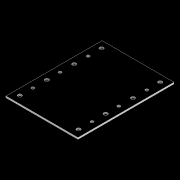
# Autodesk Inventor part: Placa
Saved by Autodesk Inventor 2020 (Build 240168000, 168)
## iProperties
Created: 2020-02-12
Part Number: Placa
Material: Generic
Document SubType Name: Modeling
Designer: PEDRO
Density: 1 g/cm^3
Appearance: Default
Author: PEDRO
Autodesk Inventor part; units mm, degrees
ref_plane "YZ Plane" through (0, 0, 0) normal (1, 0, 0) x (0, 1, 0)
ref_plane "XZ Plane" through (0, 0, 0) normal (0, 1, 0) x (-1, 0, 0)
ref_plane "XY Plane" through (0, 0, 0) normal (0, 0, 1) x (1, 0, 0)
sketch "Sketch1" plane through (0, 0, 0) normal (0, 1, 0) x (-1, 0, 0)
  line L0 (0, 0) -> (75, 0)
  line L1 (75, 0) -> (75, -100)
  line L2 (75, -100) -> (0, -100)
  line L3 (0, -100) -> (0, 0)
  circle A0 centre (68.28, -7.71) radius 2
  circle A1 centre (68.28, -35.95) radius 2
  circle A2 centre (68.28, -64.35) radius 2
  circle A3 centre (68.28, -92.9) radius 2
  circle A4 centre (7.12, -7.71) radius 2
  circle A5 centre (7.12, -35.95) radius 2
  circle A6 centre (7.12, -64.4) radius 2
  circle A7 centre (7.12, -92.8) radius 2
  circle A8 centre (7.12, -21.73) radius 1.5
  circle A9 centre (7.12, -49.67) radius 1.5
  circle A10 centre (7.12, -78.83) radius 1.5
  circle A11 centre (68.28, -21.28) radius 1.5
  circle A12 centre (68.28, -49.62) radius 1.5
  circle A13 centre (68.28, -78.83) radius 1.5
  line L4 (68.28, 0) -> (68.28, -100) construction
  line L5 (7.12, 0) -> (7.12, -100) construction
  dimension "d0" = 75
  dimension "d1" = 100
  dimension "d2" = 7.12
  dimension "d3" = 6.72
  dimension "d4" = 4
  dimension "d5" = 3
  dimension "d6" = 4
  dimension "d7" = 3
  dimension "d8" = 4
  dimension "d9" = 3
  dimension "d10" = 4
  dimension "d11" = 4
  dimension "d12" = 3
  dimension "d13" = 4
  dimension "d14" = 3
  dimension "d15" = 4
  dimension "d16" = 3
  dimension "d17" = 4
  dimension "d18" = 7.71
  dimension "d19" = 21.73
  dimension "d20" = 35.95
  dimension "d21" = 49.67
  dimension "d22" = 64.4
  dimension "d23" = 78.83
  dimension "d24" = 92.8
  dimension "d25" = 7.71
  dimension "d26" = 21.28
  dimension "d27" = 35.95
  dimension "d28" = 49.62
  dimension "d29" = 64.35
  dimension "d30" = 78.83
  dimension "d31" = 92.9
  constraints: 14 centre point, 8 end point, 4 point on line, 2 horizontal, 2 parallel, 1 perpendicular, 20 other
  measures "d0" distance of L1.end L2.end
  measures "d1" distance of L0.end L1.end
  measures "d4" diameter of A3
  measures "d5" diameter of A13
  measures "d6" diameter of A2
  measures "d7" diameter of A12
  measures "d8" diameter of A1
  measures "d9" diameter of A11
  measures "d10" diameter of A0
  measures "d11" diameter of A4
  measures "d12" diameter of A8
  measures "d13" diameter of A5
  measures "d14" diameter of A9
  measures "d15" diameter of A6
  measures "d16" diameter of A10
  measures "d17" diameter of A7
  measures "d18" distance from line of L0 A4.centre
  measures "d19" distance from line of L0 A8.centre
  measures "d20" distance from line of L0 A5.centre
  measures "d21" distance from line of L0 A9.centre
  measures "d22" distance from line of L0 A6.centre
  measures "d23" distance from line of L0 A10.centre
  measures "d24" distance from line of L0 A7.centre
  measures "d25" distance from line of L0 A0.centre
  measures "d26" distance from line of L0 A11.centre
  measures "d27" distance from line of L0 A1.centre
  measures "d28" distance from line of L0 A12.centre
  measures "d29" distance from line of L0 A2.centre
  measures "d30" distance from line of L0 A13.centre
  measures "d31" distance from line of L0 A3.centre
extrude "Extrusion1" add sketch "Sketch1" along normal blind 1.6
body "Solid1"
